Autodesk Inventor part; units mm, degrees
(part 5 of 6)
  line L3563 (-18.9253, -22.4708) -> (-19.0757, -22.5683)
  line L3564 (-19.0757, -22.5683) -> (-19.2381, -22.6688)
  line L3565 (-19.2381, -22.6688) -> (-19.4148, -22.773)
  line L3566 (-19.4148, -22.773) -> (-19.6036, -22.8791)
  line L3567 (-19.6036, -22.8791) -> (-19.8047, -22.9867)
  line L3568 (-19.8047, -22.9867) -> (-20.0203, -23.0963)
  line L3569 (-20.0203, -23.0963) -> (-20.2484, -23.2063)
  line L3570 (-20.2484, -23.2063) -> (-20.4495, -23.2985)
  arc A110 (-21.0333, -22.7728) -> (-20.4495, -23.2985) centre (0, 0) ccw
  line L3571 (-21.0333, -22.7728) -> (-20.9626, -22.5632)
  line L3572 (-20.9626, -22.5632) -> (-20.8771, -22.3249)
  line L3573 (-20.8771, -22.3249) -> (-20.7906, -22.099)
  line L3574 (-20.7906, -22.099) -> (-20.7047, -21.8877)
  line L3575 (-20.7047, -21.8877) -> (-20.6189, -21.6889)
  line L3576 (-20.6189, -21.6889) -> (-20.5336, -21.5022)
  line L3577 (-20.5336, -21.5022) -> (-20.4507, -21.3302)
  line L3578 (-20.4507, -21.3302) -> (-20.3695, -21.1705)
  line L3579 (-20.3695, -21.1705) -> (-20.2025, -20.8614)
  line L3580 (-20.2025, -20.8614) -> (-20.1865, -20.8174)
  line L3581 (-20.1865, -20.8174) -> (-20.181, -20.7821)
  line L3582 (-20.181, -20.7821) -> (-20.1856, -20.7559)
  line L3583 (-20.1856, -20.7559) -> (-20.1955, -20.7424)
  line L3584 (-20.1955, -20.7424) -> (-20.4707, -20.4707)
  line L3585 (-20.4707, -20.4707) -> (-20.7424, -20.1955)
  line L3586 (-20.7424, -20.1955) -> (-20.7559, -20.1856)
  line L3587 (-20.7559, -20.1856) -> (-20.7821, -20.181)
  line L3588 (-20.7821, -20.181) -> (-20.8174, -20.1865)
  line L3589 (-20.8174, -20.1865) -> (-20.8614, -20.2025)
  line L3590 (-20.8614, -20.2025) -> (-21.1705, -20.3695)
  line L3591 (-21.1705, -20.3695) -> (-21.3302, -20.4507)
  line L3592 (-21.3302, -20.4507) -> (-21.5022, -20.5336)
  line L3593 (-21.5022, -20.5336) -> (-21.6889, -20.6189)
  line L3594 (-21.6889, -20.6189) -> (-21.8877, -20.7047)
  line L3595 (-21.8877, -20.7047) -> (-22.099, -20.7906)
  line L3596 (-22.099, -20.7906) -> (-22.3249, -20.8771)
  line L3597 (-22.3249, -20.8771) -> (-22.5632, -20.9626)
  line L3598 (-22.5632, -20.9626) -> (-22.7728, -21.0333)
  arc A111 (-23.2985, -20.4495) -> (-22.7728, -21.0333) centre (0, 0) ccw
  line L3599 (-23.2985, -20.4495) -> (-23.2063, -20.2484)
  line L3600 (-23.2063, -20.2484) -> (-23.0963, -20.0203)
  line L3601 (-23.0963, -20.0203) -> (-22.9867, -19.8047)
  line L3602 (-22.9867, -19.8047) -> (-22.8791, -19.6036)
  line L3603 (-22.8791, -19.6036) -> (-22.773, -19.4148)
  line L3604 (-22.773, -19.4148) -> (-22.6688, -19.2381)
  line L3605 (-22.6688, -19.2381) -> (-22.5683, -19.0757)
  line L3606 (-22.5683, -19.0757) -> (-22.4708, -18.9253)
  line L3607 (-22.4708, -18.9253) -> (-22.2724, -18.6353)
  line L3608 (-22.2724, -18.6353) -> (-22.2519, -18.5933)
  line L3609 (-22.2519, -18.5933) -> (-22.2427, -18.5587)
  line L3610 (-22.2427, -18.5587) -> (-22.2446, -18.5322)
  line L3611 (-22.2446, -18.5322) -> (-22.2531, -18.5178)
  line L3612 (-22.2531, -18.5178) -> (-22.4984, -18.2188)
  line L3613 (-22.4984, -18.2188) -> (-22.7398, -17.9167)
  line L3614 (-22.7398, -17.9167) -> (-22.7521, -17.9055)
  line L3615 (-22.7521, -17.9055) -> (-22.7777, -17.8981)
  line L3616 (-22.7777, -17.8981) -> (-22.8134, -17.8999)
  line L3617 (-22.8134, -17.8999) -> (-22.8588, -17.9112)
  line L3618 (-22.8588, -17.9112) -> (-23.1837, -18.045)
  line L3619 (-23.1837, -18.045) -> (-23.3511, -18.1091)
  line L3620 (-23.3511, -18.1091) -> (-23.5308, -18.1736)
  line L3621 (-23.5308, -18.1736) -> (-23.7253, -18.2388)
  line L3622 (-23.7253, -18.2388) -> (-23.932, -18.3034)
  line L3623 (-23.932, -18.3034) -> (-24.1511, -18.3668)
  line L3624 (-24.1511, -18.3668) -> (-24.3848, -18.4292)
  line L3625 (-24.3848, -18.4292) -> (-24.6308, -18.4893)
  line L3626 (-24.6308, -18.4893) -> (-24.8466, -18.5377)
  arc A112 (-25.3084, -17.9021) -> (-24.8466, -18.5377) centre (0, 0) ccw
  line L3627 (-25.3084, -17.9021) -> (-25.1957, -17.7118)
  line L3628 (-25.1957, -17.7118) -> (-25.0625, -17.4964)
  line L3629 (-25.0625, -17.4964) -> (-24.931, -17.2934)
  line L3630 (-24.931, -17.2934) -> (-24.8029, -17.1047)
  line L3631 (-24.8029, -17.1047) -> (-24.6777, -16.928)
  line L3632 (-24.6777, -16.928) -> (-24.5555, -16.7632)
  line L3633 (-24.5555, -16.7632) -> (-24.4386, -16.6122)
  line L3634 (-24.4386, -16.6122) -> (-24.326, -16.4728)
  line L3635 (-24.326, -16.4728) -> (-24.0984, -16.2052)
  line L3636 (-24.0984, -16.2052) -> (-24.0735, -16.1655)
  line L3637 (-24.0735, -16.1655) -> (-24.0608, -16.1321)
  line L3638 (-24.0608, -16.1321) -> (-24.0599, -16.1055)
  line L3639 (-24.0599, -16.1055) -> (-24.0668, -16.0903)
  line L3640 (-24.0668, -16.0903) -> (-24.2795, -15.7673)
  line L3641 (-24.2795, -15.7673) -> (-24.488, -15.4416)
  line L3642 (-24.488, -15.4416) -> (-24.4991, -15.4291)
  line L3643 (-24.4991, -15.4291) -> (-24.5238, -15.4191)
  line L3644 (-24.5238, -15.4191) -> (-24.5595, -15.4172)
  line L3645 (-24.5595, -15.4172) -> (-24.6058, -15.4237)
  line L3646 (-24.6058, -15.4237) -> (-24.9429, -15.5228)
  line L3647 (-24.9429, -15.5228) -> (-25.1161, -15.569)
  line L3648 (-25.1161, -15.569) -> (-25.3015, -15.6144)
  line L3649 (-25.3015, -15.6144) -> (-25.5018, -15.6589)
  line L3650 (-25.5018, -15.6589) -> (-25.7142, -15.7015)
  line L3651 (-25.7142, -15.7015) -> (-25.9387, -15.7417)
  line L3652 (-25.9387, -15.7417) -> (-26.1776, -15.7793)
  line L3653 (-26.1776, -15.7793) -> (-26.4285, -15.8134)
  line L3654 (-26.4285, -15.8134) -> (-26.6482, -15.8389)
  arc A113 (-27.041, -15.1586) -> (-26.6482, -15.8389) centre (0, 0) ccw
  line L3655 (-27.041, -15.1586) -> (-26.9091, -14.9811)
  line L3656 (-26.9091, -14.9811) -> (-26.7541, -14.7808)
  line L3657 (-26.7541, -14.7808) -> (-26.602, -14.5927)
  line L3658 (-26.602, -14.5927) -> (-26.455, -14.4184)
  line L3659 (-26.455, -14.4184) -> (-26.312, -14.2558)
  line L3660 (-26.312, -14.2558) -> (-26.1732, -14.1046)
  line L3661 (-26.1732, -14.1046) -> (-26.0412, -13.9666)
  line L3662 (-26.0412, -13.9666) -> (-25.9146, -13.8398)
  line L3663 (-25.9146, -13.8398) -> (-25.6603, -13.5974)
  line L3664 (-25.6603, -13.5974) -> (-25.6314, -13.5605)
  line L3665 (-25.6314, -13.5605) -> (-25.6153, -13.5287)
  line L3666 (-25.6153, -13.5287) -> (-25.6116, -13.5023)
  line L3667 (-25.6116, -13.5023) -> (-25.6168, -13.4865)
  line L3668 (-25.6168, -13.4865) -> (-25.7946, -13.143)
  line L3669 (-25.7946, -13.143) -> (-25.968, -12.7973)
  line L3670 (-25.968, -12.7973) -> (-25.9777, -12.7837)
  line L3671 (-25.9777, -12.7837) -> (-26.0012, -12.7712)
  line L3672 (-26.0012, -12.7712) -> (-26.0365, -12.7656)
  line L3673 (-26.0365, -12.7656) -> (-26.0833, -12.7672)
  line L3674 (-26.0833, -12.7672) -> (-26.4288, -12.8305)
  line L3675 (-26.4288, -12.8305) -> (-26.6059, -12.8584)
  line L3676 (-26.6059, -12.8584) -> (-26.7951, -12.8841)
  line L3677 (-26.7951, -12.8841) -> (-26.9989, -12.9075)
  line L3678 (-26.9989, -12.9075) -> (-27.2145, -12.9276)
  line L3679 (-27.2145, -12.9276) -> (-27.442, -12.9441)
  line L3680 (-27.442, -12.9441) -> (-27.6836, -12.9565)
  line L3681 (-27.6836, -12.9565) -> (-27.9367, -12.9642)
  line L3682 (-27.9367, -12.9642) -> (-28.1579, -12.9667)
  arc A114 (-28.4774, -12.249) -> (-28.1579, -12.9667) centre (0, 0) ccw
  line L3683 (-28.4774, -12.249) -> (-28.3276, -12.0862)
  line L3684 (-28.3276, -12.0862) -> (-28.1525, -11.9033)
  line L3685 (-28.1525, -11.9033) -> (-27.9817, -11.7321)
  line L3686 (-27.9817, -11.7321) -> (-27.8172, -11.5741)
  line L3687 (-27.8172, -11.5741) -> (-27.6579, -11.4273)
  line L3688 (-27.6579, -11.4273) -> (-27.5042, -11.2915)
  line L3689 (-27.5042, -11.2915) -> (-27.3584, -11.1681)
  line L3690 (-27.3584, -11.1681) -> (-27.2193, -11.0551)
  line L3691 (-27.2193, -11.0551) -> (-26.941, -10.8407)
  line L3692 (-26.941, -10.8407) -> (-26.9085, -10.807)
  line L3693 (-26.9085, -10.807) -> (-26.8891, -10.777)
  line L3694 (-26.8891, -10.777) -> (-26.8826, -10.7512)
  line L3695 (-26.8826, -10.7512) -> (-26.8862, -10.7349)
  line L3696 (-26.8862, -10.7349) -> (-27.0272, -10.3748)
  line L3697 (-27.0272, -10.3748) -> (-27.1634, -10.0128)
  line L3698 (-27.1634, -10.0128) -> (-27.1717, -9.9983)
  line L3699 (-27.1717, -9.9983) -> (-27.1937, -9.9834)
  line L3700 (-27.1937, -9.9834) -> (-27.2282, -9.9741)
  line L3701 (-27.2282, -9.9741) -> (-27.2749, -9.9708)
  line L3702 (-27.2749, -9.9708) -> (-27.6252, -9.9977)
  line L3703 (-27.6252, -9.9977) -> (-27.8042, -10.0069)
  line L3704 (-27.8042, -10.0069) -> (-27.995, -10.0127)
  line L3705 (-27.995, -10.0127) -> (-28.2002, -10.0146)
  line L3706 (-28.2002, -10.0146) -> (-28.4168, -10.0121)
  line L3707 (-28.4168, -10.0121) -> (-28.6447, -10.0047)
  line L3708 (-28.6447, -10.0047) -> (-28.8863, -9.9918)
  line L3709 (-28.8863, -9.9918) -> (-29.1388, -9.973)
  line L3710 (-29.1388, -9.973) -> (-29.359, -9.9523)
  arc A115 (-29.6018, -9.2052) -> (-29.359, -9.9523) centre (0, 0) ccw
  line L3711 (-29.6018, -9.2052) -> (-29.4358, -9.059)
  line L3712 (-29.4358, -9.059) -> (-29.2425, -8.8954)
  line L3713 (-29.2425, -8.8954) -> (-29.0547, -8.7429)
  line L3714 (-29.0547, -8.7429) -> (-28.8746, -8.603)
  line L3715 (-28.8746, -8.603) -> (-28.7009, -8.4737)
  line L3716 (-28.7009, -8.4737) -> (-28.5338, -8.3547)
  line L3717 (-28.5338, -8.3547) -> (-28.3759, -8.2472)
  line L3718 (-28.3759, -8.2472) -> (-28.2257, -8.1494)
  line L3719 (-28.2257, -8.1494) -> (-27.9266, -7.9652)
  line L3720 (-27.9266, -7.9652) -> (-27.8907, -7.9351)
  line L3721 (-27.8907, -7.9351) -> (-27.8683, -7.9073)
  line L3722 (-27.8683, -7.9073) -> (-27.8592, -7.8823)
  line L3723 (-27.8592, -7.8823) -> (-27.861, -7.8657)
  line L3724 (-27.861, -7.8657) -> (-27.9636, -7.4928)
  line L3725 (-27.9636, -7.4928) -> (-28.0612, -7.1186)
  line L3726 (-28.0612, -7.1186) -> (-28.0679, -7.1033)
  line L3727 (-28.0679, -7.1033) -> (-28.0883, -7.0862)
  line L3728 (-28.0883, -7.0862) -> (-28.1216, -7.0733)
  line L3729 (-28.1216, -7.0733) -> (-28.1677, -7.0652)
  line L3730 (-28.1677, -7.0652) -> (-28.5189, -7.0553)
  line L3731 (-28.5189, -7.0553) -> (-28.6979, -7.0457)
  line L3732 (-28.6979, -7.0457) -> (-28.8883, -7.0315)
  line L3733 (-28.8883, -7.0315) -> (-29.0926, -7.012)
  line L3734 (-29.0926, -7.012) -> (-29.3077, -6.9869)
  line L3735 (-29.3077, -6.9869) -> (-29.5336, -6.9557)
  line L3736 (-29.5336, -6.9557) -> (-29.7725, -6.9177)
  line L3737 (-29.7725, -6.9177) -> (-30.0216, -6.8726)
  line L3738 (-30.0216, -6.8726) -> (-30.2385, -6.829)
  arc A116 (-30.4018, -6.0605) -> (-30.2385, -6.829) centre (0, 0) ccw
  line L3739 (-30.4018, -6.0605) -> (-30.2214, -5.9325)
  line L3740 (-30.2214, -5.9325) -> (-30.0122, -5.79)
  line L3741 (-30.0122, -5.79) -> (-29.8094, -5.658)
  line L3742 (-29.8094, -5.658) -> (-29.6157, -5.5376)
  line L3743 (-29.6157, -5.5376) -> (-29.4294, -5.4272)
  line L3744 (-29.4294, -5.4272) -> (-29.2508, -5.3263)
  line L3745 (-29.2508, -5.3263) -> (-29.0826, -5.2359)
  line L3746 (-29.0826, -5.2359) -> (-28.9229, -5.1544)
  line L3747 (-28.9229, -5.1544) -> (-28.6062, -5.0025)
  line L3748 (-28.6062, -5.0025) -> (-28.5674, -4.9763)
  line L3749 (-28.5674, -4.9763) -> (-28.5421, -4.951)
  line L3750 (-28.5421, -4.951) -> (-28.5305, -4.927)
  line L3751 (-28.5305, -4.927) -> (-28.5306, -4.9104)
  line L3752 (-28.5306, -4.9104) -> (-28.5936, -4.5288)
  line L3753 (-28.5936, -4.5288) -> (-28.6516, -4.1464)
  line L3754 (-28.6516, -4.1464) -> (-28.6567, -4.1305)
  line L3755 (-28.6567, -4.1305) -> (-28.6751, -4.1114)
  line L3756 (-28.6751, -4.1114) -> (-28.7069, -4.0951)
  line L3757 (-28.7069, -4.0951) -> (-28.7519, -4.0822)
  line L3758 (-28.7519, -4.0822) -> (-29.1001, -4.0356)
  line L3759 (-29.1001, -4.0356) -> (-29.2771, -4.0074)
  line L3760 (-29.2771, -4.0074) -> (-29.465, -3.9734)
  line L3761 (-29.465, -3.9734) -> (-29.6661, -3.9326)
  line L3762 (-29.6661, -3.9326) -> (-29.8774, -3.8852)
  line L3763 (-29.8774, -3.8852) -> (-30.0989, -3.8305)
  line L3764 (-30.0989, -3.8305) -> (-30.3325, -3.7677)
  line L3765 (-30.3325, -3.7677) -> (-30.5755, -3.6968)
  line L3766 (-30.5755, -3.6968) -> (-30.7866, -3.6308)
  arc A117 (-30.8688, -2.8495) -> (-30.7866, -3.6308) centre (0, 0) ccw
  line L3767 (-30.8688, -2.8495) -> (-30.676, -2.741)
  line L3768 (-30.676, -2.741) -> (-30.453, -2.6211)
  line L3769 (-30.453, -2.6211) -> (-30.2376, -2.5111)
  line L3770 (-30.2376, -2.5111) -> (-30.0323, -2.4116)
  line L3771 (-30.0323, -2.4116) -> (-29.8355, -2.3213)
  line L3772 (-29.8355, -2.3213) -> (-29.6473, -2.2396)
  line L3773 (-29.6473, -2.2396) -> (-29.4705, -2.1673)
  line L3774 (-29.4705, -2.1673) -> (-29.3033, -2.1029)
  line L3775 (-29.3033, -2.1029) -> (-28.9724, -1.9849)
  line L3776 (-28.9724, -1.9849) -> (-28.931, -1.9629)
  line L3777 (-28.931, -1.9629) -> (-28.9033, -1.9404)
  line L3778 (-28.9033, -1.9404) -> (-28.8892, -1.9178)
  line L3779 (-28.8892, -1.9178) -> (-28.8876, -1.9012)
  line L3780 (-28.8876, -1.9012) -> (-28.9103, -1.5151)
  line L3781 (-28.9103, -1.5151) -> (-28.9281, -1.1288)
  line L3782 (-28.9281, -1.1288) -> (-28.9314, -1.1124)
  line L3783 (-28.9314, -1.1124) -> (-28.9478, -1.0915)
  line L3784 (-28.9478, -1.0915) -> (-28.9777, -1.0719)
  line L3785 (-28.9777, -1.0719) -> (-29.0211, -1.0544)
  line L3786 (-29.0211, -1.0544) -> (-29.3626, -0.9717)
  line L3787 (-29.3626, -0.9717) -> (-29.5356, -0.9251)
  line L3788 (-29.5356, -0.9251) -> (-29.719, -0.8717)
  line L3789 (-29.719, -0.8717) -> (-29.9147, -0.8101)
  line L3790 (-29.9147, -0.8101) -> (-30.1199, -0.7408)
  line L3791 (-30.1199, -0.7408) -> (-30.3344, -0.6634)
  line L3792 (-30.3344, -0.6634) -> (-30.5601, -0.5765)
  line L3793 (-30.5601, -0.5765) -> (-30.7945, -0.4805)
  line L3794 (-30.7945, -0.4805) -> (-30.9975, -0.3928)
  arc A118 (-30.9975, 0.3928) -> (-30.9975, -0.3928) centre (0, 0) ccw
  line L3795 (-30.9975, 0.3928) -> (-30.7945, 0.4805)
  line L3796 (-30.7945, 0.4805) -> (-30.5601, 0.5765)
  line L3797 (-30.5601, 0.5765) -> (-30.3344, 0.6634)
  line L3798 (-30.3344, 0.6634) -> (-30.1199, 0.7408)
  line L3799 (-30.1199, 0.7408) -> (-29.9147, 0.8101)
  line L3800 (-29.9147, 0.8101) -> (-29.719, 0.8717)
  line L3801 (-29.719, 0.8717) -> (-29.5356, 0.9251)
  line L3802 (-29.5356, 0.9251) -> (-29.3626, 0.9717)
  line L3803 (-29.3626, 0.9717) -> (-29.0211, 1.0544)
  line L3804 (-29.0211, 1.0544) -> (-28.9777, 1.0719)
  line L3805 (-28.9777, 1.0719) -> (-28.9478, 1.0915)
  line L3806 (-28.9478, 1.0915) -> (-28.9314, 1.1124)
  line L3807 (-28.9314, 1.1124) -> (-28.9281, 1.1288)
  line L3808 (-28.9281, 1.1288) -> (-28.9103, 1.5151)
  line L3809 (-28.9103, 1.5151) -> (-28.8876, 1.9012)
  line L3810 (-28.8876, 1.9012) -> (-28.8892, 1.9178)
  line L3811 (-28.8892, 1.9178) -> (-28.9033, 1.9404)
  line L3812 (-28.9033, 1.9404) -> (-28.931, 1.9629)
  line L3813 (-28.931, 1.9629) -> (-28.9724, 1.9849)
  line L3814 (-28.9724, 1.9849) -> (-29.3033, 2.1029)
  line L3815 (-29.3033, 2.1029) -> (-29.4705, 2.1673)
  line L3816 (-29.4705, 2.1673) -> (-29.6473, 2.2396)
  line L3817 (-29.6473, 2.2396) -> (-29.8355, 2.3213)
  line L3818 (-29.8355, 2.3213) -> (-30.0323, 2.4116)
  line L3819 (-30.0323, 2.4116) -> (-30.2376, 2.5111)
  line L3820 (-30.2376, 2.5111) -> (-30.453, 2.6211)
  line L3821 (-30.453, 2.6211) -> (-30.676, 2.741)
  line L3822 (-30.676, 2.741) -> (-30.8688, 2.8495)
  arc A119 (-30.7866, 3.6308) -> (-30.8688, 2.8495) centre (0, 0) ccw
  line L3823 (-30.7866, 3.6308) -> (-30.5755, 3.6968)
  line L3824 (-30.5755, 3.6968) -> (-30.3325, 3.7677)
  line L3825 (-30.3325, 3.7677) -> (-30.0989, 3.8305)
  line L3826 (-30.0989, 3.8305) -> (-29.8774, 3.8852)
  line L3827 (-29.8774, 3.8852) -> (-29.6661, 3.9326)
  line L3828 (-29.6661, 3.9326) -> (-29.465, 3.9734)
  line L3829 (-29.465, 3.9734) -> (-29.2771, 4.0074)
  line L3830 (-29.2771, 4.0074) -> (-29.1001, 4.0356)
  line L3831 (-29.1001, 4.0356) -> (-28.7519, 4.0822)
  line L3832 (-28.7519, 4.0822) -> (-28.7069, 4.0951)
  line L3833 (-28.7069, 4.0951) -> (-28.6751, 4.1114)
  line L3834 (-28.6751, 4.1114) -> (-28.6567, 4.1305)
  line L3835 (-28.6567, 4.1305) -> (-28.6516, 4.1464)
  line L3836 (-28.6516, 4.1464) -> (-28.5936, 4.5288)
  line L3837 (-28.5936, 4.5288) -> (-28.5306, 4.9104)
  line L3838 (-28.5306, 4.9104) -> (-28.5305, 4.927)
  line L3839 (-28.5305, 4.927) -> (-28.5421, 4.951)
  line L3840 (-28.5421, 4.951) -> (-28.5674, 4.9763)
  line L3841 (-28.5674, 4.9763) -> (-28.6062, 5.0025)
  line L3842 (-28.6062, 5.0025) -> (-28.9229, 5.1544)
  line L3843 (-28.9229, 5.1544) -> (-29.0826, 5.2359)
  line L3844 (-29.0826, 5.2359) -> (-29.2508, 5.3263)
  line L3845 (-29.2508, 5.3263) -> (-29.4294, 5.4272)
  line L3846 (-29.4294, 5.4272) -> (-29.6157, 5.5376)
  line L3847 (-29.6157, 5.5376) -> (-29.8094, 5.658)
  line L3848 (-29.8094, 5.658) -> (-30.0122, 5.79)
  line L3849 (-30.0122, 5.79) -> (-30.2214, 5.9325)
  line L3850 (-30.2214, 5.9325) -> (-30.4018, 6.0605)
  arc A120 (-30.2385, 6.829) -> (-30.4018, 6.0605) centre (0, 0) ccw
  line L3851 (-30.2385, 6.829) -> (-30.0216, 6.8726)
  line L3852 (-30.0216, 6.8726) -> (-29.7725, 6.9177)
  line L3853 (-29.7725, 6.9177) -> (-29.5336, 6.9557)
  line L3854 (-29.5336, 6.9557) -> (-29.3077, 6.9869)
  line L3855 (-29.3077, 6.9869) -> (-29.0926, 7.012)
  line L3856 (-29.0926, 7.012) -> (-28.8883, 7.0315)
  line L3857 (-28.8883, 7.0315) -> (-28.6979, 7.0457)
  line L3858 (-28.6979, 7.0457) -> (-28.5189, 7.0553)
  line L3859 (-28.5189, 7.0553) -> (-28.1677, 7.0652)
  line L3860 (-28.1677, 7.0652) -> (-28.1216, 7.0733)
  line L3861 (-28.1216, 7.0733) -> (-28.0883, 7.0862)
  line L3862 (-28.0883, 7.0862) -> (-28.0679, 7.1033)
  line L3863 (-28.0679, 7.1033) -> (-28.0612, 7.1186)
  line L3864 (-28.0612, 7.1186) -> (-27.9636, 7.4928)
  line L3865 (-27.9636, 7.4928) -> (-27.861, 7.8657)
  line L3866 (-27.861, 7.8657) -> (-27.8592, 7.8823)
  line L3867 (-27.8592, 7.8823) -> (-27.8683, 7.9073)
  line L3868 (-27.8683, 7.9073) -> (-27.8907, 7.9351)
  line L3869 (-27.8907, 7.9351) -> (-27.9266, 7.9652)
  line L3870 (-27.9266, 7.9652) -> (-28.2257, 8.1494)
  line L3871 (-28.2257, 8.1494) -> (-28.3759, 8.2472)
  line L3872 (-28.3759, 8.2472) -> (-28.5338, 8.3547)
  line L3873 (-28.5338, 8.3547) -> (-28.7009, 8.4737)
  line L3874 (-28.7009, 8.4737) -> (-28.8746, 8.603)
  line L3875 (-28.8746, 8.603) -> (-29.0547, 8.7429)
  line L3876 (-29.0547, 8.7429) -> (-29.2425, 8.8954)
  line L3877 (-29.2425, 8.8954) -> (-29.4358, 9.059)
  line L3878 (-29.4358, 9.059) -> (-29.6018, 9.2052)
  arc A121 (-29.359, 9.9523) -> (-29.6018, 9.2052) centre (0, 0) ccw
  line L3879 (-29.359, 9.9523) -> (-29.1388, 9.973)
  line L3880 (-29.1388, 9.973) -> (-28.8863, 9.9918)
  line L3881 (-28.8863, 9.9918) -> (-28.6447, 10.0047)
  line L3882 (-28.6447, 10.0047) -> (-28.4168, 10.0121)
  line L3883 (-28.4168, 10.0121) -> (-28.2002, 10.0146)
  line L3884 (-28.2002, 10.0146) -> (-27.995, 10.0127)
  line L3885 (-27.995, 10.0127) -> (-27.8042, 10.0069)
  line L3886 (-27.8042, 10.0069) -> (-27.6252, 9.9977)
  line L3887 (-27.6252, 9.9977) -> (-27.2749, 9.9708)
  line L3888 (-27.2749, 9.9708) -> (-27.2282, 9.9741)
  line L3889 (-27.2282, 9.9741) -> (-27.1937, 9.9834)
  line L3890 (-27.1937, 9.9834) -> (-27.1717, 9.9983)
  line L3891 (-27.1717, 9.9983) -> (-27.1634, 10.0128)
  line L3892 (-27.1634, 10.0128) -> (-27.0272, 10.3748)
  line L3893 (-27.0272, 10.3748) -> (-26.8862, 10.7349)
  line L3894 (-26.8862, 10.7349) -> (-26.8826, 10.7512)
  line L3895 (-26.8826, 10.7512) -> (-26.8891, 10.777)
  line L3896 (-26.8891, 10.777) -> (-26.9085, 10.807)
  line L3897 (-26.9085, 10.807) -> (-26.941, 10.8407)
  line L3898 (-26.941, 10.8407) -> (-27.2193, 11.0551)
  line L3899 (-27.2193, 11.0551) -> (-27.3584, 11.1681)
  line L3900 (-27.3584, 11.1681) -> (-27.5042, 11.2915)
  line L3901 (-27.5042, 11.2915) -> (-27.6579, 11.4273)
  line L3902 (-27.6579, 11.4273) -> (-27.8172, 11.5741)
  line L3903 (-27.8172, 11.5741) -> (-27.9817, 11.7321)
  line L3904 (-27.9817, 11.7321) -> (-28.1525, 11.9033)
  line L3905 (-28.1525, 11.9033) -> (-28.3276, 12.0862)
  line L3906 (-28.3276, 12.0862) -> (-28.4774, 12.249)
  arc A122 (-28.1579, 12.9667) -> (-28.4774, 12.249) centre (0, 0) ccw
  line L3907 (-28.1579, 12.9667) -> (-27.9367, 12.9642)
  line L3908 (-27.9367, 12.9642) -> (-27.6836, 12.9565)
  line L3909 (-27.6836, 12.9565) -> (-27.442, 12.9441)
  line L3910 (-27.442, 12.9441) -> (-27.2145, 12.9276)
  line L3911 (-27.2145, 12.9276) -> (-26.9989, 12.9075)
  line L3912 (-26.9989, 12.9075) -> (-26.7951, 12.8841)
  line L3913 (-26.7951, 12.8841) -> (-26.6059, 12.8584)
  line L3914 (-26.6059, 12.8584) -> (-26.4288, 12.8305)
  line L3915 (-26.4288, 12.8305) -> (-26.0833, 12.7672)
  line L3916 (-26.0833, 12.7672) -> (-26.0365, 12.7656)
  line L3917 (-26.0365, 12.7656) -> (-26.0012, 12.7712)
  line L3918 (-26.0012, 12.7712) -> (-25.9777, 12.7837)
  line L3919 (-25.9777, 12.7837) -> (-25.968, 12.7973)
  line L3920 (-25.968, 12.7973) -> (-25.7946, 13.143)
  line L3921 (-25.7946, 13.143) -> (-25.6168, 13.4865)
  line L3922 (-25.6168, 13.4865) -> (-25.6116, 13.5023)
  line L3923 (-25.6116, 13.5023) -> (-25.6153, 13.5287)
  line L3924 (-25.6153, 13.5287) -> (-25.6314, 13.5605)
  line L3925 (-25.6314, 13.5605) -> (-25.6603, 13.5974)
  line L3926 (-25.6603, 13.5974) -> (-25.9146, 13.8398)
  line L3927 (-25.9146, 13.8398) -> (-26.0412, 13.9666)
  line L3928 (-26.0412, 13.9666) -> (-26.1732, 14.1046)
  line L3929 (-26.1732, 14.1046) -> (-26.312, 14.2558)
  line L3930 (-26.312, 14.2558) -> (-26.455, 14.4184)
  line L3931 (-26.455, 14.4184) -> (-26.602, 14.5927)
  line L3932 (-26.602, 14.5927) -> (-26.7541, 14.7808)
  line L3933 (-26.7541, 14.7808) -> (-26.9091, 14.9811)
  line L3934 (-26.9091, 14.9811) -> (-27.041, 15.1586)
  arc A123 (-26.6482, 15.8389) -> (-27.041, 15.1586) centre (0, 0) ccw
  line L3935 (-26.6482, 15.8389) -> (-26.4285, 15.8134)
  line L3936 (-26.4285, 15.8134) -> (-26.1776, 15.7793)
  line L3937 (-26.1776, 15.7793) -> (-25.9387, 15.7417)
  line L3938 (-25.9387, 15.7417) -> (-25.7142, 15.7015)
  line L3939 (-25.7142, 15.7015) -> (-25.5018, 15.6589)
  line L3940 (-25.5018, 15.6589) -> (-25.3015, 15.6144)
  line L3941 (-25.3015, 15.6144) -> (-25.1161, 15.569)
  line L3942 (-25.1161, 15.569) -> (-24.9429, 15.5228)
  line L3943 (-24.9429, 15.5228) -> (-24.6058, 15.4237)
  line L3944 (-24.6058, 15.4237) -> (-24.5595, 15.4172)
  line L3945 (-24.5595, 15.4172) -> (-24.5238, 15.4191)
  line L3946 (-24.5238, 15.4191) -> (-24.4991, 15.4291)
  line L3947 (-24.4991, 15.4291) -> (-24.488, 15.4416)
  line L3948 (-24.488, 15.4416) -> (-24.2795, 15.7673)
  line L3949 (-24.2795, 15.7673) -> (-24.0668, 16.0903)
  line L3950 (-24.0668, 16.0903) -> (-24.0599, 16.1055)
  line L3951 (-24.0599, 16.1055) -> (-24.0608, 16.1321)
  line L3952 (-24.0608, 16.1321) -> (-24.0735, 16.1655)
  line L3953 (-24.0735, 16.1655) -> (-24.0984, 16.2052)
  line L3954 (-24.0984, 16.2052) -> (-24.326, 16.4728)
  line L3955 (-24.326, 16.4728) -> (-24.4386, 16.6122)
  line L3956 (-24.4386, 16.6122) -> (-24.5555, 16.7632)
  line L3957 (-24.5555, 16.7632) -> (-24.6777, 16.928)
  line L3958 (-24.6777, 16.928) -> (-24.8029, 17.1047)
  line L3959 (-24.8029, 17.1047) -> (-24.931, 17.2934)
  line L3960 (-24.931, 17.2934) -> (-25.0625, 17.4964)
  line L3961 (-25.0625, 17.4964) -> (-25.1957, 17.7118)
  line L3962 (-25.1957, 17.7118) -> (-25.3084, 17.9021)
  arc A124 (-24.8466, 18.5377) -> (-25.3084, 17.9021) centre (0, 0) ccw
  line L3963 (-24.8466, 18.5377) -> (-24.6308, 18.4893)
  line L3964 (-24.6308, 18.4893) -> (-24.3848, 18.4292)
  line L3965 (-24.3848, 18.4292) -> (-24.1511, 18.3668)
  line L3966 (-24.1511, 18.3668) -> (-23.932, 18.3034)
  line L3967 (-23.932, 18.3034) -> (-23.7253, 18.2388)
  line L3968 (-23.7253, 18.2388) -> (-23.5308, 18.1736)
  line L3969 (-23.5308, 18.1736) -> (-23.3511, 18.1091)
  line L3970 (-23.3511, 18.1091) -> (-23.1837, 18.045)
  line L3971 (-23.1837, 18.045) -> (-22.8588, 17.9112)
  line L3972 (-22.8588, 17.9112) -> (-22.8134, 17.8999)
  line L3973 (-22.8134, 17.8999) -> (-22.7777, 17.8981)
  line L3974 (-22.7777, 17.8981) -> (-22.7521, 17.9055)
  line L3975 (-22.7521, 17.9055) -> (-22.7398, 17.9167)
  line L3976 (-22.7398, 17.9167) -> (-22.4984, 18.2188)
  line L3977 (-22.4984, 18.2188) -> (-22.2531, 18.5178)
  line L3978 (-22.2531, 18.5178) -> (-22.2446, 18.5322)
  line L3979 (-22.2446, 18.5322) -> (-22.2427, 18.5587)
  line L3980 (-22.2427, 18.5587) -> (-22.2519, 18.5933)
  line L3981 (-22.2519, 18.5933) -> (-22.2724, 18.6353)
  line L3982 (-22.2724, 18.6353) -> (-22.4708, 18.9253)
  line L3983 (-22.4708, 18.9253) -> (-22.5683, 19.0757)
  line L3984 (-22.5683, 19.0757) -> (-22.6688, 19.2381)
  line L3985 (-22.6688, 19.2381) -> (-22.773, 19.4148)
  line L3986 (-22.773, 19.4148) -> (-22.8791, 19.6036)
  line L3987 (-22.8791, 19.6036) -> (-22.9867, 19.8047)
  line L3988 (-22.9867, 19.8047) -> (-23.0963, 20.0203)
  line L3989 (-23.0963, 20.0203) -> (-23.2063, 20.2484)
  line L3990 (-23.2063, 20.2484) -> (-23.2985, 20.4495)
  arc A125 (-22.7728, 21.0333) -> (-23.2985, 20.4495) centre (0, 0) ccw
  line L3991 (-22.7728, 21.0333) -> (-22.5632, 20.9626)
  line L3992 (-22.5632, 20.9626) -> (-22.3249, 20.8771)
  line L3993 (-22.3249, 20.8771) -> (-22.099, 20.7906)
  line L3994 (-22.099, 20.7906) -> (-21.8877, 20.7047)
  line L3995 (-21.8877, 20.7047) -> (-21.6889, 20.6189)
  line L3996 (-21.6889, 20.6189) -> (-21.5022, 20.5336)
  line L3997 (-21.5022, 20.5336) -> (-21.3302, 20.4507)
  line L3998 (-21.3302, 20.4507) -> (-21.1705, 20.3695)
  line L3999 (-21.1705, 20.3695) -> (-20.8614, 20.2025)
  line L4000 (-20.8614, 20.2025) -> (-20.8174, 20.1865)
  line L4001 (-20.8174, 20.1865) -> (-20.7821, 20.181)
  line L4002 (-20.7821, 20.181) -> (-20.7559, 20.1856)
  line L4003 (-20.7559, 20.1856) -> (-20.7424, 20.1955)
  line L4004 (-20.7424, 20.1955) -> (-20.4707, 20.4707)
  line L4005 (-20.4707, 20.4707) -> (-20.1955, 20.7424)
  line L4006 (-20.1955, 20.7424) -> (-20.1856, 20.7559)
  line L4007 (-20.1856, 20.7559) -> (-20.181, 20.7821)
  line L4008 (-20.181, 20.7821) -> (-20.1865, 20.8174)
  line L4009 (-20.1865, 20.8174) -> (-20.2025, 20.8614)
  line L4010 (-20.2025, 20.8614) -> (-20.3695, 21.1705)
  line L4011 (-20.3695, 21.1705) -> (-20.4507, 21.3302)
  line L4012 (-20.4507, 21.3302) -> (-20.5336, 21.5022)
  line L4013 (-20.5336, 21.5022) -> (-20.6189, 21.6889)
  line L4014 (-20.6189, 21.6889) -> (-20.7047, 21.8877)
  line L4015 (-20.7047, 21.8877) -> (-20.7906, 22.099)
  line L4016 (-20.7906, 22.099) -> (-20.8771, 22.3249)
  line L4017 (-20.8771, 22.3249) -> (-20.9626, 22.5632)
  line L4018 (-20.9626, 22.5632) -> (-21.0333, 22.7728)
  arc A126 (-20.4495, 23.2985) -> (-21.0333, 22.7728) centre (0, 0) ccw
  line L4019 (-20.4495, 23.2985) -> (-20.2484, 23.2063)
  line L4020 (-20.2484, 23.2063) -> (-20.0203, 23.0963)
  line L4021 (-20.0203, 23.0963) -> (-19.8047, 22.9867)
  line L4022 (-19.8047, 22.9867) -> (-19.6036, 22.8791)
  line L4023 (-19.6036, 22.8791) -> (-19.4148, 22.773)
  line L4024 (-19.4148, 22.773) -> (-19.2381, 22.6688)
  line L4025 (-19.2381, 22.6688) -> (-19.0757, 22.5683)
  line L4026 (-19.0757, 22.5683) -> (-18.9253, 22.4708)
  line L4027 (-18.9253, 22.4708) -> (-18.6353, 22.2724)
  line L4028 (-18.6353, 22.2724) -> (-18.5933, 22.2519)
  line L4029 (-18.5933, 22.2519) -> (-18.5587, 22.2427)
  line L4030 (-18.5587, 22.2427) -> (-18.5322, 22.2446)
  line L4031 (-18.5322, 22.2446) -> (-18.5178, 22.2531)
  line L4032 (-18.5178, 22.2531) -> (-18.2188, 22.4984)
  line L4033 (-18.2188, 22.4984) -> (-17.9167, 22.7398)
  line L4034 (-17.9167, 22.7398) -> (-17.9055, 22.7521)
  line L4035 (-17.9055, 22.7521) -> (-17.8981, 22.7777)
  line L4036 (-17.8981, 22.7777) -> (-17.8999, 22.8134)
  line L4037 (-17.8999, 22.8134) -> (-17.9112, 22.8588)
  line L4038 (-17.9112, 22.8588) -> (-18.045, 23.1837)
  line L4039 (-18.045, 23.1837) -> (-18.1091, 23.3511)
  line L4040 (-18.1091, 23.3511) -> (-18.1736, 23.5308)
  line L4041 (-18.1736, 23.5308) -> (-18.2388, 23.7253)
  line L4042 (-18.2388, 23.7253) -> (-18.3034, 23.932)
  line L4043 (-18.3034, 23.932) -> (-18.3668, 24.1511)
  line L4044 (-18.3668, 24.1511) -> (-18.4292, 24.3848)
  line L4045 (-18.4292, 24.3848) -> (-18.4893, 24.6308)
  line L4046 (-18.4893, 24.6308) -> (-18.5377, 24.8466)
  arc A127 (-17.9021, 25.3084) -> (-18.5377, 24.8466) centre (0, 0) ccw
  line L4047 (-17.9021, 25.3084) -> (-17.7118, 25.1957)
  line L4048 (-17.7118, 25.1957) -> (-17.4964, 25.0625)
  line L4049 (-17.4964, 25.0625) -> (-17.2934, 24.931)
  line L4050 (-17.2934, 24.931) -> (-17.1047, 24.8029)
  line L4051 (-17.1047, 24.8029) -> (-16.928, 24.6777)
  line L4052 (-16.928, 24.6777) -> (-16.7632, 24.5555)
  line L4053 (-16.7632, 24.5555) -> (-16.6122, 24.4386)
  line L4054 (-16.6122, 24.4386) -> (-16.4728, 24.326)
  line L4055 (-16.4728, 24.326) -> (-16.2052, 24.0984)
  line L4056 (-16.2052, 24.0984) -> (-16.1655, 24.0735)
  line L4057 (-16.1655, 24.0735) -> (-16.1321, 24.0608)
  line L4058 (-16.1321, 24.0608) -> (-16.1055, 24.0599)
  line L4059 (-16.1055, 24.0599) -> (-16.0903, 24.0668)
  line L4060 (-16.0903, 24.0668) -> (-15.7673, 24.2795)
  line L4061 (-15.7673, 24.2795) -> (-15.4416, 24.488)
  line L4062 (-15.4416, 24.488) -> (-15.4291, 24.4991)
  line L4063 (-15.4291, 24.4991) -> (-15.4191, 24.5238)
  line L4064 (-15.4191, 24.5238) -> (-15.4172, 24.5595)
  line L4065 (-15.4172, 24.5595) -> (-15.4237, 24.6058)
  line L4066 (-15.4237, 24.6058) -> (-15.5228, 24.9429)
  line L4067 (-15.5228, 24.9429) -> (-15.569, 25.1161)
  line L4068 (-15.569, 25.1161) -> (-15.6144, 25.3015)
  line L4069 (-15.6144, 25.3015) -> (-15.6589, 25.5018)
  line L4070 (-15.6589, 25.5018) -> (-15.7015, 25.7142)
  line L4071 (-15.7015, 25.7142) -> (-15.7417, 25.9387)
  line L4072 (-15.7417, 25.9387) -> (-15.7793, 26.1776)
  line L4073 (-15.7793, 26.1776) -> (-15.8134, 26.4285)
  line L4074 (-15.8134, 26.4285) -> (-15.8389, 26.6482)
  arc A128 (-15.1586, 27.041) -> (-15.8389, 26.6482) centre (0, 0) ccw
  line L4075 (-15.1586, 27.041) -> (-14.9811, 26.9091)
  line L4076 (-14.9811, 26.9091) -> (-14.7808, 26.7541)
  line L4077 (-14.7808, 26.7541) -> (-14.5927, 26.602)
  line L4078 (-14.5927, 26.602) -> (-14.4184, 26.455)
  line L4079 (-14.4184, 26.455) -> (-14.2558, 26.312)
  line L4080 (-14.2558, 26.312) -> (-14.1046, 26.1732)
  line L4081 (-14.1046, 26.1732) -> (-13.9666, 26.0412)
  line L4082 (-13.9666, 26.0412) -> (-13.8398, 25.9146)
  line L4083 (-13.8398, 25.9146) -> (-13.5974, 25.6603)
  line L4084 (-13.5974, 25.6603) -> (-13.5605, 25.6314)
  line L4085 (-13.5605, 25.6314) -> (-13.5287, 25.6153)
  line L4086 (-13.5287, 25.6153) -> (-13.5023, 25.6116)
  line L4087 (-13.5023, 25.6116) -> (-13.4865, 25.6168)
  line L4088 (-13.4865, 25.6168) -> (-13.143, 25.7946)
  line L4089 (-13.143, 25.7946) -> (-12.7973, 25.968)
  line L4090 (-12.7973, 25.968) -> (-12.7837, 25.9777)
  line L4091 (-12.7837, 25.9777) -> (-12.7712, 26.0012)
  line L4092 (-12.7712, 26.0012) -> (-12.7656, 26.0365)
  line L4093 (-12.7656, 26.0365) -> (-12.7672, 26.0833)
  line L4094 (-12.7672, 26.0833) -> (-12.8305, 26.4288)
  line L4095 (-12.8305, 26.4288) -> (-12.8584, 26.6059)
  line L4096 (-12.8584, 26.6059) -> (-12.8841, 26.7951)
  line L4097 (-12.8841, 26.7951) -> (-12.9075, 26.9989)
  line L4098 (-12.9075, 26.9989) -> (-12.9276, 27.2145)
  line L4099 (-12.9276, 27.2145) -> (-12.9441, 27.442)
  line L4100 (-12.9441, 27.442) -> (-12.9565, 27.6836)
  line L4101 (-12.9565, 27.6836) -> (-12.9642, 27.9367)
  line L4102 (-12.9642, 27.9367) -> (-12.9667, 28.1579)
  arc A129 (-12.249, 28.4774) -> (-12.9667, 28.1579) centre (0, 0) ccw
  line L4103 (-12.249, 28.4774) -> (-12.0862, 28.3276)
  line L4104 (-12.0862, 28.3276) -> (-11.9033, 28.1525)
  line L4105 (-11.9033, 28.1525) -> (-11.7321, 27.9817)
  line L4106 (-11.7321, 27.9817) -> (-11.5741, 27.8172)
  line L4107 (-11.5741, 27.8172) -> (-11.4273, 27.6579)
  line L4108 (-11.4273, 27.6579) -> (-11.2915, 27.5042)
  line L4109 (-11.2915, 27.5042) -> (-11.1681, 27.3584)
  line L4110 (-11.1681, 27.3584) -> (-11.0551, 27.2193)
  line L4111 (-11.0551, 27.2193) -> (-10.8407, 26.941)
  line L4112 (-10.8407, 26.941) -> (-10.807, 26.9085)
  line L4113 (-10.807, 26.9085) -> (-10.777, 26.8891)
  line L4114 (-10.777, 26.8891) -> (-10.7512, 26.8826)
  line L4115 (-10.7512, 26.8826) -> (-10.7349, 26.8862)
  line L4116 (-10.7349, 26.8862) -> (-10.3748, 27.0272)
  line L4117 (-10.3748, 27.0272) -> (-10.0128, 27.1634)
  line L4118 (-10.0128, 27.1634) -> (-9.9983, 27.1717)
  line L4119 (-9.9983, 27.1717) -> (-9.9834, 27.1937)
  line L4120 (-9.9834, 27.1937) -> (-9.9741, 27.2282)
  line L4121 (-9.9741, 27.2282) -> (-9.9708, 27.2749)
  line L4122 (-9.9708, 27.2749) -> (-9.9977, 27.6252)
  line L4123 (-9.9977, 27.6252) -> (-10.0069, 27.8042)
  line L4124 (-10.0069, 27.8042) -> (-10.0127, 27.995)
  line L4125 (-10.0127, 27.995) -> (-10.0146, 28.2002)
  line L4126 (-10.0146, 28.2002) -> (-10.0121, 28.4168)
  line L4127 (-10.0121, 28.4168) -> (-10.0047, 28.6447)
  line L4128 (-10.0047, 28.6447) -> (-9.9918, 28.8863)
  line L4129 (-9.9918, 28.8863) -> (-9.973, 29.1388)
  line L4130 (-9.973, 29.1388) -> (-9.9523, 29.359)
  arc A130 (-9.2052, 29.6018) -> (-9.9523, 29.359) centre (0, 0) ccw
  line L4131 (-9.2052, 29.6018) -> (-9.059, 29.4358)
  line L4132 (-9.059, 29.4358) -> (-8.8954, 29.2425)
  line L4133 (-8.8954, 29.2425) -> (-8.7429, 29.0547)
  line L4134 (-8.7429, 29.0547) -> (-8.603, 28.8746)
  line L4135 (-8.603, 28.8746) -> (-8.4737, 28.7009)
  line L4136 (-8.4737, 28.7009) -> (-8.3547, 28.5338)
  line L4137 (-8.3547, 28.5338) -> (-8.2472, 28.3759)
  line L4138 (-8.2472, 28.3759) -> (-8.1494, 28.2257)
  line L4139 (-8.1494, 28.2257) -> (-7.9652, 27.9266)
  line L4140 (-7.9652, 27.9266) -> (-7.9351, 27.8907)
  line L4141 (-7.9351, 27.8907) -> (-7.9073, 27.8683)
  line L4142 (-7.9073, 27.8683) -> (-7.8823, 27.8592)
  line L4143 (-7.8823, 27.8592) -> (-7.8657, 27.861)
  line L4144 (-7.8657, 27.861) -> (-7.4928, 27.9636)
  line L4145 (-7.4928, 27.9636) -> (-7.1186, 28.0612)
  line L4146 (-7.1186, 28.0612) -> (-7.1033, 28.0679)
  line L4147 (-7.1033, 28.0679) -> (-7.0862, 28.0883)
  line L4148 (-7.0862, 28.0883) -> (-7.0733, 28.1216)
  line L4149 (-7.0733, 28.1216) -> (-7.0652, 28.1677)
  line L4150 (-7.0652, 28.1677) -> (-7.0553, 28.5189)
  line L4151 (-7.0553, 28.5189) -> (-7.0457, 28.6979)
  line L4152 (-7.0457, 28.6979) -> (-7.0315, 28.8883)
  line L4153 (-7.0315, 28.8883) -> (-7.012, 29.0926)
  line L4154 (-7.012, 29.0926) -> (-6.9869, 29.3077)
  line L4155 (-6.9869, 29.3077) -> (-6.9557, 29.5336)
  line L4156 (-6.9557, 29.5336) -> (-6.9177, 29.7725)
  line L4157 (-6.9177, 29.7725) -> (-6.8726, 30.0216)
  line L4158 (-6.8726, 30.0216) -> (-6.829, 30.2385)
  arc A131 (-6.0605, 30.4018) -> (-6.829, 30.2385) centre (0, 0) ccw
  line L4159 (-6.0605, 30.4018) -> (-5.9325, 30.2214)
  line L4160 (-5.9325, 30.2214) -> (-5.79, 30.0122)
  line L4161 (-5.79, 30.0122) -> (-5.658, 29.8094)
  line L4162 (-5.658, 29.8094) -> (-5.5376, 29.6157)
  line L4163 (-5.5376, 29.6157) -> (-5.4272, 29.4294)
  line L4164 (-5.4272, 29.4294) -> (-5.3263, 29.2508)
  line L4165 (-5.3263, 29.2508) -> (-5.2359, 29.0826)
  line L4166 (-5.2359, 29.0826) -> (-5.1544, 28.9229)
  line L4167 (-5.1544, 28.9229) -> (-5.0025, 28.6062)
  line L4168 (-5.0025, 28.6062) -> (-4.9763, 28.5674)
  line L4169 (-4.9763, 28.5674) -> (-4.951, 28.5421)
  line L4170 (-4.951, 28.5421) -> (-4.927, 28.5305)
  line L4171 (-4.927, 28.5305) -> (-4.9104, 28.5306)
  line L4172 (-4.9104, 28.5306) -> (-4.5288, 28.5936)
  line L4173 (-4.5288, 28.5936) -> (-4.1464, 28.6516)
  line L4174 (-4.1464, 28.6516) -> (-4.1305, 28.6567)
  line L4175 (-4.1305, 28.6567) -> (-4.1114, 28.6751)
  line L4176 (-4.1114, 28.6751) -> (-4.0951, 28.7069)
  line L4177 (-4.0951, 28.7069) -> (-4.0822, 28.7519)
  line L4178 (-4.0822, 28.7519) -> (-4.0356, 29.1001)
  line L4179 (-4.0356, 29.1001) -> (-4.0074, 29.2771)
  line L4180 (-4.0074, 29.2771) -> (-3.9734, 29.465)
  line L4181 (-3.9734, 29.465) -> (-3.9326, 29.6661)
  line L4182 (-3.9326, 29.6661) -> (-3.8852, 29.8774)
  line L4183 (-3.8852, 29.8774) -> (-3.8305, 30.0989)
  line L4184 (-3.8305, 30.0989) -> (-3.7677, 30.3325)
  line L4185 (-3.7677, 30.3325) -> (-3.6968, 30.5755)
  line L4186 (-3.6968, 30.5755) -> (-3.6308, 30.7866)
  arc A132 (-2.8495, 30.8688) -> (-3.6308, 30.7866) centre (0, 0) ccw
  line L4187 (-2.8495, 30.8688) -> (-2.741, 30.676)
  line L4188 (-2.741, 30.676) -> (-2.6211, 30.453)
  line L4189 (-2.6211, 30.453) -> (-2.5111, 30.2376)
  line L4190 (-2.5111, 30.2376) -> (-2.4116, 30.0323)
  line L4191 (-2.4116, 30.0323) -> (-2.3213, 29.8355)
  line L4192 (-2.3213, 29.8355) -> (-2.2396, 29.6473)
  line L4193 (-2.2396, 29.6473) -> (-2.1673, 29.4705)
  line L4194 (-2.1673, 29.4705) -> (-2.1029, 29.3033)
  line L4195 (-2.1029, 29.3033) -> (-1.9849, 28.9724)
  line L4196 (-1.9849, 28.9724) -> (-1.9629, 28.931)
  line L4197 (-1.9629, 28.931) -> (-1.9404, 28.9033)
  line L4198 (-1.9404, 28.9033) -> (-1.9178, 28.8892)
  line L4199 (-1.9178, 28.8892) -> (-1.9012, 28.8876)
  line L4200 (-1.9012, 28.8876) -> (-1.5151, 28.9103)
  line L4201 (-1.5151, 28.9103) -> (-1.1288, 28.9281)
  line L4202 (-1.1288, 28.9281) -> (-1.1124, 28.9314)
  line L4203 (-1.1124, 28.9314) -> (-1.0915, 28.9478)
  line L4204 (-1.0915, 28.9478) -> (-1.0719, 28.9777)
  line L4205 (-1.0719, 28.9777) -> (-1.0544, 29.0211)
  line L4206 (-1.0544, 29.0211) -> (-0.9717, 29.3626)
  line L4207 (-0.9717, 29.3626) -> (-0.9251, 29.5356)
  line L4208 (-0.9251, 29.5356) -> (-0.8717, 29.719)
  line L4209 (-0.8717, 29.719) -> (-0.8101, 29.9147)
  line L4210 (-0.8101, 29.9147) -> (-0.7408, 30.1199)
  line L4211 (-0.7408, 30.1199) -> (-0.6634, 30.3344)
  line L4212 (-0.6634, 30.3344) -> (-0.5765, 30.5601)
  line L4213 (-0.5765, 30.5601) -> (-0.4805, 30.7945)
  line L4214 (-0.4805, 30.7945) -> (-0.3928, 30.9975)
  arc A133 (0.3928, 30.9975) -> (-0.3928, 30.9975) centre (0, 0) ccw
  line L4215 (0.3928, 30.9975) -> (0.4805, 30.7945)
  line L4216 (0.4805, 30.7945) -> (0.5765, 30.5601)
  line L4217 (0.5765, 30.5601) -> (0.6634, 30.3344)
  line L4218 (0.6634, 30.3344) -> (0.7408, 30.1199)
  line L4219 (0.7408, 30.1199) -> (0.8101, 29.9147)
  line L4220 (0.8101, 29.9147) -> (0.8717, 29.719)
  line L4221 (0.8717, 29.719) -> (0.9251, 29.5356)
  line L4222 (0.9251, 29.5356) -> (0.9717, 29.3626)
  line L4223 (0.9717, 29.3626) -> (1.0544, 29.0211)
  line L4224 (1.0544, 29.0211) -> (1.0719, 28.9777)
  line L4225 (1.0719, 28.9777) -> (1.0915, 28.9478)
  line L4226 (1.0915, 28.9478) -> (1.1124, 28.9314)
  line L4227 (1.1124, 28.9314) -> (1.1288, 28.9281)
  line L4228 (1.1288, 28.9281) -> (1.5151, 28.9103)
  line L4229 (1.5151, 28.9103) -> (1.9012, 28.8876)
  line L4230 (1.9012, 28.8876) -> (1.9178, 28.8892)
  line L4231 (1.9178, 28.8892) -> (1.9404, 28.9033)
  line L4232 (1.9404, 28.9033) -> (1.9629, 28.931)
  line L4233 (1.9629, 28.931) -> (1.9849, 28.9724)
  line L4234 (1.9849, 28.9724) -> (2.1029, 29.3033)
  line L4235 (2.1029, 29.3033) -> (2.1673, 29.4705)
  line L4236 (2.1673, 29.4705) -> (2.2396, 29.6473)
  line L4237 (2.2396, 29.6473) -> (2.3213, 29.8355)
  line L4238 (2.3213, 29.8355) -> (2.4116, 30.0323)
  line L4239 (2.4116, 30.0323) -> (2.5111, 30.2376)
  line L4240 (2.5111, 30.2376) -> (2.6211, 30.453)
  line L4241 (2.6211, 30.453) -> (2.741, 30.676)
  line L4242 (2.741, 30.676) -> (2.8495, 30.8688)
  arc A134 (3.6308, 30.7866) -> (2.8495, 30.8688) centre (0, 0) ccw
  line L4243 (3.6308, 30.7866) -> (3.6968, 30.5755)
  line L4244 (3.6968, 30.5755) -> (3.7677, 30.3325)
  line L4245 (3.7677, 30.3325) -> (3.8305, 30.0989)
  line L4246 (3.8305, 30.0989) -> (3.8852, 29.8774)
  line L4247 (3.8852, 29.8774) -> (3.9326, 29.6661)
  line L4248 (3.9326, 29.6661) -> (3.9734, 29.465)
  line L4249 (3.9734, 29.465) -> (4.0074, 29.2771)
  line L4250 (4.0074, 29.2771) -> (4.0356, 29.1001)
  line L4251 (4.0356, 29.1001) -> (4.0822, 28.7519)
  line L4252 (4.0822, 28.7519) -> (4.0951, 28.7069)
  line L4253 (4.0951, 28.7069) -> (4.1114, 28.6751)
  line L4254 (4.1114, 28.6751) -> (4.1305, 28.6567)
  line L4255 (4.1305, 28.6567) -> (4.1464, 28.6516)
  line L4256 (4.1464, 28.6516) -> (4.5288, 28.5936)
  line L4257 (4.5288, 28.5936) -> (4.9104, 28.5306)
  line L4258 (4.9104, 28.5306) -> (4.927, 28.5305)
  line L4259 (4.927, 28.5305) -> (4.951, 28.5421)
  line L4260 (4.951, 28.5421) -> (4.9763, 28.5674)
  line L4261 (4.9763, 28.5674) -> (5.0025, 28.6062)
  line L4262 (5.0025, 28.6062) -> (5.1544, 28.9229)
  line L4263 (5.1544, 28.9229) -> (5.2359, 29.0826)
  line L4264 (5.2359, 29.0826) -> (5.3263, 29.2508)
  line L4265 (5.3263, 29.2508) -> (5.4272, 29.4294)
  line L4266 (5.4272, 29.4294) -> (5.5376, 29.6157)
  line L4267 (5.5376, 29.6157) -> (5.658, 29.8094)
  line L4268 (5.658, 29.8094) -> (5.79, 30.0122)
  line L4269 (5.79, 30.0122) -> (5.9325, 30.2214)
  line L4270 (5.9325, 30.2214) -> (6.0605, 30.4018)
  arc A135 (6.829, 30.2385) -> (6.0605, 30.4018) centre (0, 0) ccw
  line L4271 (6.829, 30.2385) -> (6.8726, 30.0216)
  line L4272 (6.8726, 30.0216) -> (6.9177, 29.7725)
  line L4273 (6.9177, 29.7725) -> (6.9557, 29.5336)
  line L4274 (6.9557, 29.5336) -> (6.9869, 29.3077)
  line L4275 (6.9869, 29.3077) -> (7.012, 29.0926)
  line L4276 (7.012, 29.0926) -> (7.0315, 28.8883)
  line L4277 (7.0315, 28.8883) -> (7.0457, 28.6979)
  line L4278 (7.0457, 28.6979) -> (7.0553, 28.5189)
  line L4279 (7.0553, 28.5189) -> (7.0652, 28.1677)
  line L4280 (7.0652, 28.1677) -> (7.0733, 28.1216)
  line L4281 (7.0733, 28.1216) -> (7.0862, 28.0883)
  line L4282 (7.0862, 28.0883) -> (7.1033, 28.0679)
  line L4283 (7.1033, 28.0679) -> (7.1186, 28.0612)
  line L4284 (7.1186, 28.0612) -> (7.4928, 27.9636)
  line L4285 (7.4928, 27.9636) -> (7.8657, 27.861)
  line L4286 (7.8657, 27.861) -> (7.8823, 27.8592)
  line L4287 (7.8823, 27.8592) -> (7.9073, 27.8683)
  line L4288 (7.9073, 27.8683) -> (7.9351, 27.8907)
  line L4289 (7.9351, 27.8907) -> (7.9652, 27.9266)
  line L4290 (7.9652, 27.9266) -> (8.1494, 28.2257)
  line L4291 (8.1494, 28.2257) -> (8.2472, 28.3759)
  line L4292 (8.2472, 28.3759) -> (8.3547, 28.5338)
  line L4293 (8.3547, 28.5338) -> (8.4737, 28.7009)
  line L4294 (8.4737, 28.7009) -> (8.603, 28.8746)
  line L4295 (8.603, 28.8746) -> (8.7429, 29.0547)
  line L4296 (8.7429, 29.0547) -> (8.8954, 29.2425)
  line L4297 (8.8954, 29.2425) -> (9.059, 29.4358)
  line L4298 (9.059, 29.4358) -> (9.2052, 29.6018)
  arc A136 (9.9523, 29.359) -> (9.2052, 29.6018) centre (0, 0) ccw
  line L4299 (9.9523, 29.359) -> (9.973, 29.1388)
  line L4300 (9.973, 29.1388) -> (9.9918, 28.8863)
  line L4301 (9.9918, 28.8863) -> (10.0047, 28.6447)
  line L4302 (10.0047, 28.6447) -> (10.0121, 28.4168)
  line L4303 (10.0121, 28.4168) -> (10.0146, 28.2002)
  line L4304 (10.0146, 28.2002) -> (10.0127, 27.995)
  line L4305 (10.0127, 27.995) -> (10.0069, 27.8042)
  line L4306 (10.0069, 27.8042) -> (9.9977, 27.6252)
  line L4307 (9.9977, 27.6252) -> (9.9708, 27.2749)
  line L4308 (9.9708, 27.2749) -> (9.9741, 27.2282)
  line L4309 (9.9741, 27.2282) -> (9.9834, 27.1937)
  line L4310 (9.9834, 27.1937) -> (9.9983, 27.1717)
  line L4311 (9.9983, 27.1717) -> (10.0128, 27.1634)
  line L4312 (10.0128, 27.1634) -> (10.3748, 27.0272)
  line L4313 (10.3748, 27.0272) -> (10.7349, 26.8862)
  line L4314 (10.7349, 26.8862) -> (10.7512, 26.8826)
  line L4315 (10.7512, 26.8826) -> (10.777, 26.8891)
  line L4316 (10.777, 26.8891) -> (10.807, 26.9085)
  line L4317 (10.807, 26.9085) -> (10.8407, 26.941)
  line L4318 (10.8407, 26.941) -> (11.0551, 27.2193)
  line L4319 (11.0551, 27.2193) -> (11.1681, 27.3584)
  line L4320 (11.1681, 27.3584) -> (11.2915, 27.5042)
  line L4321 (11.2915, 27.5042) -> (11.4273, 27.6579)
  line L4322 (11.4273, 27.6579) -> (11.5741, 27.8172)
  line L4323 (11.5741, 27.8172) -> (11.7321, 27.9817)
  line L4324 (11.7321, 27.9817) -> (11.9033, 28.1525)
  line L4325 (11.9033, 28.1525) -> (12.0862, 28.3276)
  line L4326 (12.0862, 28.3276) -> (12.249, 28.4774)
  arc A137 (12.9667, 28.1579) -> (12.249, 28.4774) centre (0, 0) ccw
  line L4327 (12.9667, 28.1579) -> (12.9642, 27.9367)
  line L4328 (12.9642, 27.9367) -> (12.9565, 27.6836)
  line L4329 (12.9565, 27.6836) -> (12.9441, 27.442)
  line L4330 (12.9441, 27.442) -> (12.9276, 27.2145)
  line L4331 (12.9276, 27.2145) -> (12.9075, 26.9989)
  line L4332 (12.9075, 26.9989) -> (12.8841, 26.7951)
  line L4333 (12.8841, 26.7951) -> (12.8584, 26.6059)
  line L4334 (12.8584, 26.6059) -> (12.8305, 26.4288)
  line L4335 (12.8305, 26.4288) -> (12.7672, 26.0833)
  line L4336 (12.7672, 26.0833) -> (12.7656, 26.0365)
  line L4337 (12.7656, 26.0365) -> (12.7712, 26.0012)
  line L4338 (12.7712, 26.0012) -> (12.7837, 25.9777)
  line L4339 (12.7837, 25.9777) -> (12.7973, 25.968)
  line L4340 (12.7973, 25.968) -> (13.143, 25.7946)
  line L4341 (13.143, 25.7946) -> (13.4865, 25.6168)
  line L4342 (13.4865, 25.6168) -> (13.5023, 25.6116)
  line L4343 (13.5023, 25.6116) -> (13.5287, 25.6153)
  line L4344 (13.5287, 25.6153) -> (13.5605, 25.6314)
  line L4345 (13.5605, 25.6314) -> (13.5974, 25.6603)
  line L4346 (13.5974, 25.6603) -> (13.8398, 25.9146)
  line L4347 (13.8398, 25.9146) -> (13.9666, 26.0412)
  line L4348 (13.9666, 26.0412) -> (14.1046, 26.1732)
  line L4349 (14.1046, 26.1732) -> (14.2558, 26.312)
  line L4350 (14.2558, 26.312) -> (14.4184, 26.455)
  line L4351 (14.4184, 26.455) -> (14.5927, 26.602)
  line L4352 (14.5927, 26.602) -> (14.7808, 26.7541)
  line L4353 (14.7808, 26.7541) -> (14.9811, 26.9091)
  line L4354 (14.9811, 26.9091) -> (15.1586, 27.041)
  arc A138 (15.8389, 26.6482) -> (15.1586, 27.041) centre (0, 0) ccw
  line L4355 (15.8389, 26.6482) -> (15.8134, 26.4285)
  line L4356 (15.8134, 26.4285) -> (15.7793, 26.1776)
  line L4357 (15.7793, 26.1776) -> (15.7417, 25.9387)
  line L4358 (15.7417, 25.9387) -> (15.7015, 25.7142)
  line L4359 (15.7015, 25.7142) -> (15.6589, 25.5018)
  line L4360 (15.6589, 25.5018) -> (15.6144, 25.3015)
  line L4361 (15.6144, 25.3015) -> (15.569, 25.1161)
  line L4362 (15.569, 25.1161) -> (15.5228, 24.9429)
  line L4363 (15.5228, 24.9429) -> (15.4237, 24.6058)
  line L4364 (15.4237, 24.6058) -> (15.4172, 24.5595)
  line L4365 (15.4172, 24.5595) -> (15.4191, 24.5238)
  line L4366 (15.4191, 24.5238) -> (15.4291, 24.4991)
  line L4367 (15.4291, 24.4991) -> (15.4416, 24.488)
  line L4368 (15.4416, 24.488) -> (15.7673, 24.2795)
  line L4369 (15.7673, 24.2795) -> (16.0903, 24.0668)
  line L4370 (16.0903, 24.0668) -> (16.1055, 24.0599)
  line L4371 (16.1055, 24.0599) -> (16.1321, 24.0608)
  line L4372 (16.1321, 24.0608) -> (16.1655, 24.0735)
  line L4373 (16.1655, 24.0735) -> (16.2052, 24.0984)
  line L4374 (16.2052, 24.0984) -> (16.4728, 24.326)
  line L4375 (16.4728, 24.326) -> (16.6122, 24.4386)
  line L4376 (16.6122, 24.4386) -> (16.7632, 24.5555)
  line L4377 (16.7632, 24.5555) -> (16.928, 24.6777)
  line L4378 (16.928, 24.6777) -> (17.1047, 24.8029)
  line L4379 (17.1047, 24.8029) -> (17.2934, 24.931)
  line L4380 (17.2934, 24.931) -> (17.4964, 25.0625)
  line L4381 (17.4964, 25.0625) -> (17.7118, 25.1957)
  line L4382 (17.7118, 25.1957) -> (17.9021, 25.3084)
  arc A139 (18.5377, 24.8466) -> (17.9021, 25.3084) centre (0, 0) ccw
  line L4383 (18.5377, 24.8466) -> (18.4893, 24.6308)
  line L4384 (18.4893, 24.6308) -> (18.4292, 24.3848)
  line L4385 (18.4292, 24.3848) -> (18.3668, 24.1511)
  line L4386 (18.3668, 24.1511) -> (18.3034, 23.932)
  line L4387 (18.3034, 23.932) -> (18.2388, 23.7253)
  line L4388 (18.2388, 23.7253) -> (18.1736, 23.5308)
  line L4389 (18.1736, 23.5308) -> (18.1091, 23.3511)
  line L4390 (18.1091, 23.3511) -> (18.045, 23.1837)
  line L4391 (18.045, 23.1837) -> (17.9112, 22.8588)
  line L4392 (17.9112, 22.8588) -> (17.8999, 22.8134)
  line L4393 (17.8999, 22.8134) -> (17.8981, 22.7777)
  line L4394 (17.8981, 22.7777) -> (17.9055, 22.7521)
  line L4395 (17.9055, 22.7521) -> (17.9167, 22.7398)
  line L4396 (17.9167, 22.7398) -> (18.2188, 22.4984)
  line L4397 (18.2188, 22.4984) -> (18.5178, 22.2531)
  line L4398 (18.5178, 22.2531) -> (18.5322, 22.2446)
  line L4399 (18.5322, 22.2446) -> (18.5587, 22.2427)
  line L4400 (18.5587, 22.2427) -> (18.5933, 22.2519)
  line L4401 (18.5933, 22.2519) -> (18.6353, 22.2724)
  line L4402 (18.6353, 22.2724) -> (18.9253, 22.4708)
  line L4403 (18.9253, 22.4708) -> (19.0757, 22.5683)
  line L4404 (19.0757, 22.5683) -> (19.2381, 22.6688)
  line L4405 (19.2381, 22.6688) -> (19.4148, 22.773)
  line L4406 (19.4148, 22.773) -> (19.6036, 22.8791)
  line L4407 (19.6036, 22.8791) -> (19.8047, 22.9867)
  line L4408 (19.8047, 22.9867) -> (20.0203, 23.0963)
  line L4409 (20.0203, 23.0963) -> (20.2484, 23.2063)
  line L4410 (20.2484, 23.2063) -> (20.4495, 23.2985)
  arc A140 (21.0333, 22.7728) -> (20.4495, 23.2985) centre (0, 0) ccw
  line L4411 (21.0333, 22.7728) -> (20.9626, 22.5632)
  line L4412 (20.9626, 22.5632) -> (20.8771, 22.3249)
  line L4413 (20.8771, 22.3249) -> (20.7906, 22.099)
  line L4414 (20.7906, 22.099) -> (20.7047, 21.8877)
  line L4415 (20.7047, 21.8877) -> (20.6189, 21.6889)
  line L4416 (20.6189, 21.6889) -> (20.5336, 21.5022)
  line L4417 (20.5336, 21.5022) -> (20.4507, 21.3302)
  line L4418 (20.4507, 21.3302) -> (20.3695, 21.1705)
  line L4419 (20.3695, 21.1705) -> (20.2025, 20.8614)
  line L4420 (20.2025, 20.8614) -> (20.1865, 20.8174)
  line L4421 (20.1865, 20.8174) -> (20.181, 20.7821)
  line L4422 (20.181, 20.7821) -> (20.1856, 20.7559)
  line L4423 (20.1856, 20.7559) -> (20.1955, 20.7424)
  line L4424 (20.1955, 20.7424) -> (20.4707, 20.4707)
  line L4425 (20.4707, 20.4707) -> (20.7424, 20.1955)
  line L4426 (20.7424, 20.1955) -> (20.7559, 20.1856)
  line L4427 (20.7559, 20.1856) -> (20.7821, 20.181)
  line L4428 (20.7821, 20.181) -> (20.8174, 20.1865)
  line L4429 (20.8174, 20.1865) -> (20.8614, 20.2025)
  line L4430 (20.8614, 20.2025) -> (21.1705, 20.3695)
  line L4431 (21.1705, 20.3695) -> (21.3302, 20.4507)
  line L4432 (21.3302, 20.4507) -> (21.5022, 20.5336)